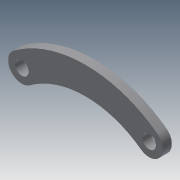
# Autodesk Inventor part: neco2
Saved by Autodesk Inventor 2013 (Build 170138000, 138)
## iProperties
Created: 2013-03-09
Part Number: neco2
Material: Generic
Document SubType Name: Modeling
Designer: idle-rug
Density: 1 g/cm^3
Author: idle-rug
Autodesk Inventor part; units mm, degrees
ref_plane "YZ Plane" through (0, 0, 0) normal (1, 0, 0) x (0, 1, 0)
ref_plane "XZ Plane" through (0, 0, 0) normal (0, 1, 0) x (-1, 0, 0)
ref_plane "XY Plane" through (0, 0, 0) normal (0, 0, 1) x (1, 0, 0)
sketch "Sketch1" plane through (0, 0, 0) normal (0, 1, 0) x (-1, 0, 0)
  circle A0 centre (-14, 0) radius 3
  circle A1 centre (14, 0) radius 3
  circle A2 centre (-14, 0) radius 1.5
  circle A3 centre (14, 0) radius 1.5
  line L0 (0, 14) -> (0, -14)
  line L1 (0, 0) -> (0, -19)
  line L2 (0, 1.6008) -> (0, 7.6008)
  arc A4 (15.7796, 2.4152) -> (-15.7796, 2.4152) centre (0, -19) ccw
  arc A5 (12.2204, -2.4152) -> (-12.2204, -2.4152) centre (0, -19) ccw
  dimension "d1" = 6
  dimension "d2" = 6
  dimension "d3" = 3
  dimension "d4" = 3
  dimension "d5" = 19
  dimension "d7" = 6
  constraints: 10 point on circle, 6 centre point, 6 end point, 3 coincident, 3 point on line, 1 vertical
  measures "d1" diameter of A0
  measures "d2" diameter of A1
  measures "d3" diameter of A2
  measures "d4" diameter of A3
  measures "d5" distance of L1.start L1.end
  measures "d7" distance of L2.start L2.end
extrude "Extrusion1" add sketch "Sketch1" along normal blind 2
body "Solid1"
